# Autodesk Inventor part: linkage
Saved by Autodesk Inventor 2014 SP1 (Build 180222100, 222)
## iProperties
Created: 2014-01-25
Part Number: linkage
Material: Generic
Document SubType Name: Modeling
Designer: tom
Density: 1 g/cm^3
Appearance: Default
Author: tom
Autodesk Inventor part; units mm, degrees
ref_plane "YZ Plane" through (0, 0, 0) normal (1, 0, 0) x (0, 1, 0)
ref_plane "XZ Plane" through (0, 0, 0) normal (0, 1, 0) x (-1, 0, 0)
ref_plane "XY Plane" through (0, 0, 0) normal (0, 0, 1) x (1, 0, 0)
sketch "Sketch1" plane through (0, 0, 0) normal (0, 0, 1) x (1, 0, 0)
  circle A0 centre (-3.2581, -3.2482) radius 0.75
  circle A1 centre (11.7419, -13.2482) radius 0.75
  arc A2 (11.7419, -16.7482) -> (11.7419, -9.7482) centre (11.7419, -13.2482) ccw
  arc A3 (0.2419, -3.2482) -> (-6.7581, -3.2482) centre (-3.2581, -3.2482) ccw
  circle A4 centre (11.7419, -13.2482) radius 0.75
  circle A5 centre (-3.2581, -3.2482) radius 0.75
  line L0 (0.2419, -3.2482) -> (0.2419, -8.2482)
  line L1 (-6.7581, -3.2482) -> (-6.7581, -10.2482)
  line L2 (11.7419, -9.7482) -> (2.2419, -9.7482)
  line L3 (2.2419, -9.7482) -> (0.2419, -8.2482)
  line L4 (11.7419, -16.7482) -> (0.2419, -16.7482)
  line L5 (-6.7581, -10.2482) -> (0.2419, -16.7482)
  point P0 (0, 0)
  point P1 (-5.7424, -0.7828)
  point P2 (9.5175, -10.546)
  dimension "d0" = 7
  dimension "d1" = 7
  dimension "d4" = 5
  dimension "d5" = 7
  dimension "d6" = 9.5
  dimension "d7" = 11.5
  dimension "d8" = 15
  constraints: 12 end point, 6 centre point, 6 point on circle, 4 coincident, 4 tangent, 2 concentric, 2 parallel, 1 perpendicular, 1 vertical
  measures "d0" diameter of A2
  measures "d1" diameter of A3
  measures "d4" distance of L0.start L0.end
  measures "d5" distance of L1.start L1.end
  measures "d6" distance of L2.start L2.end
  measures "d7" distance of L4.start L4.end
  measures "d8" horizontal distance of A0.centre A1.centre
extrude "Extrusion1" add sketch "Sketch1" against normal blind 4
body "Solid1"
